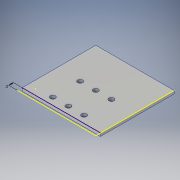
# Autodesk Inventor part: nhk20
Saved by Autodesk Inventor 2019 (Build 230136000, 136)
## iProperties
Created: 2022-02-15
Part Number: nhk20
Material: アルミニウム 6061
Document SubType Name: Sheet Metal
Designer: yuta
Density: 2.7 g/cm^3
Sheet Metal Rule: Default_mm
Appearance: アルミニウム - フラット
Mass: 12.461 g
Surface Area: 51.1627 cm^2
Volume: 4.61518 cm^3
Author: yuta
Autodesk Inventor part; units mm, degrees
ref_plane "YZ Plane" through (0, 0, 0) normal (1, 0, 0) x (0, 1, 0)
ref_plane "XZ Plane" through (0, 0, 0) normal (0, 1, 0) x (-1, 0, 0)
ref_plane "XY Plane" through (0, 0, 0) normal (0, 0, 1) x (1, 0, 0)
sketch "スケッチ1" plane through (0, 0, 0) normal (0, 1, 0) x (-1, 0, 0)
  line L0 (5.0263, 6.4044) -> (-44.9737, 6.4044)
  line L1 (-44.9737, 6.4044) -> (-44.9737, -43.5956)
  line L2 (-44.9737, -43.5956) -> (5.0263, -43.5956)
  line L3 (5.0263, -43.5956) -> (5.0263, 6.4044)
  point P0 (0, 0)
  dimension "d0" = 50
  dimension "d1" = 50
  constraints: 8 end point, 2 parallel, 1 horizontal, 1 perpendicular
  measures "d0" distance of L2.end L1.end
  measures "d1" distance of L1.end L0.end
extrude "押し出し1" add sketch "スケッチ1" along normal blind 2
sketch "スケッチ2" plane through (0, 2, 0) normal (0, 1, 0) x (1, 0, 0)
  circle A0 centre (19.9737, 1.0956) radius 1.5
  line L0 (-5.0263, -6.4044) -> (44.9737, -6.4044) projected
  line L1 (-5.0263, 43.5956) -> (-5.0263, -6.4044) projected
  circle A1 centre (9.9737, 1.0956) radius 1.5
  circle A2 centre (29.9737, 1.0956) radius 1.5
  circle A3 centre (9.9737, 18.5956) radius 1.5
  circle A4 centre (19.9737, 18.5956) radius 1.5
  circle A5 centre (29.9737, 18.5956) radius 1.5
  point P0 (0, 0)
  dimension "d4" = 3
  dimension "d5" = 7.5
  dimension "d6" = 25
  dimension "d7" = 3
  dimension "d8" = 3
  dimension "d9" = 10
  dimension "d10" = 10
  dimension "d11" = 3
  dimension "d12" = 17.5
  dimension "d13" = 3
  dimension "d14" = 3
  dimension "d15" = 10
  dimension "d16" = 10
  dimension "d17" = 17.5
  constraints: 6 centre point
  measures "d4" diameter of A0
  measures "d5" distance from line of A0.centre L0
  measures "d6" distance from line of L1 A0.centre
  measures "d7" diameter of A1
  measures "d8" diameter of A2
  measures "d9" distance of A1.centre A0.centre
  measures "d10" distance of A2.centre A0.centre
  measures "d11" diameter of A3
  measures "d12" distance of A1.centre A3.centre
  measures "d13" diameter of A4
  measures "d14" diameter of A5
  measures "d15" distance of A4.centre A3.centre
  measures "d16" distance of A5.centre A4.centre
  measures "d17" distance of A2.centre A5.centre
hole "穴1" at (9.9737, 2, -1.0956) at (19.9737, 2, -1.0956) at (29.9737, 2, -1.0956) at (9.9737, 2, -18.5956) at (19.9737, 2, -18.5956) at (29.9737, 2, -18.5956) direction (0, -1, 0) diameter 3 depth 2
sketch "スケッチ3" plane through (0, 2, 0) normal (0, 1, 0) x (1, 0, 0)
  line L0 (-4.9253, -3.4044) -> (44.9737, -3.4044)
  line L1 (44.9737, -6.4044) -> (44.9737, 43.5956) projected
  line L2 (-5.0263, -6.4044) -> (44.9737, -6.4044) projected
  point P0 (0, 0)
  dimension "d25" = 3
  constraints: 2 end point, 1 horizontal, 1 point on line
  measures "d25" distance between parallel lines of L2 L0
sketch "スケッチ4" plane through (0, 2, 0) normal (0, 1, 0) x (1, 0, 0)
  line L0 (-5.0263, 43.5956) -> (-5.0263, -6.4044) projected
  line L1 (-5.0263, -6.4044) -> (44.9737, -6.4044) projected
  line L2 (-5.0263, -6.4044) -> (44.9737, -6.4044)
  line L3 (44.9737, -6.4044) -> (44.9737, -3.4044)
  line L4 (44.9737, -6.4044) -> (44.9737, 43.5956) projected
  line L5 (44.9737, -3.4044) -> (-5.0263, -3.4044)
  line L6 (-5.0263, -3.4044) -> (-5.0263, -6.4044)
  point P0 (0, 0)
  dimension "d26" = 3
  constraints: 8 end point, 2 perpendicular, 1 horizontal, 1 point on line
  measures "d26" distance of L1.end L3.end
extrude "押し出し2" cut sketch "スケッチ4" against normal blind 10
sketch "スケッチ5" plane through (0, 2, 0) normal (0, 1, 0) x (1, 0, 0)
  circle A0 centre (9.9737, 1.0956) radius 1.6
  line L0 (-5.0263, -3.4044) -> (44.9737, -3.4044) projected
  circle A1 centre (9.9737, 18.5956) radius 1.5 projected
  circle A2 centre (9.9737, 18.5956) radius 1.6
  circle A3 centre (19.9737, 18.5956) radius 1.6
  circle A4 centre (19.9737, 1.0956) radius 1.6
  circle A5 centre (29.9737, 18.5956) radius 1.6
  circle A6 centre (29.9737, 1.0956) radius 1.6
  line L1 (-5.0263, 43.5956) -> (-5.0263, -3.4044) projected
  point P0 (0, 0)
  dimension "d29" = 3.2
  dimension "d30" = 4.5
  dimension "d32" = 3.2
  dimension "d33" = 3.2
  dimension "d34" = 3.2
  dimension "d35" = 3.2
  dimension "d36" = 3.2
  dimension "d37" = 4.5
  dimension "d38" = 17.5
  dimension "d39" = 17.5
  dimension "d40" = 17.5
  dimension "d41" = 4.5
  dimension "d42" = 10
  dimension "d43" = 10
  dimension "d44" = 10
  dimension "d45" = 15
  dimension "d46" = 15
  dimension "d47" = 10
  constraints: 6 centre point, 1 coincident
  measures "d29" diameter of A0
  measures "d30" distance from line of L0 A0.centre
  measures "d32" diameter of A2
  measures "d33" diameter of A3
  measures "d34" diameter of A4
  measures "d35" diameter of A5
  measures "d36" diameter of A6
  measures "d37" distance from line of L0 A4.centre
  measures "d38" distance of A1.centre A0.centre
  measures "d39" distance of A4.centre A3.centre
  measures "d40" distance of A6.centre A5.centre
  measures "d41" distance from line of L0 A6.centre
  measures "d42" distance of A3.centre A1.centre
  measures "d43" distance of A5.centre A3.centre
  measures "d44" distance of A4.centre A0.centre
  measures "d45" distance from line of L1 A1.centre
  measures "d46" distance from line of L1 A0.centre
  measures "d47" distance of A4.centre A6.centre
hole "穴2" at (9.9737, 2, -1.0956) at (19.9737, 2, -1.0956) at (29.9737, 2, -1.0956) at (29.9737, 2, -18.5956) at (19.9737, 2, -18.5956) at (9.9737, 2, -18.5956) direction (0, -1, 0) diameter 3.2 depth 3
equation "\"BendRadius\" = Thickness"
equation "\"BendReliefWidth\" = Thickness"
equation "\"BendReliefDepth\" = 0.5 * Thickness"
equation "\"CornerReliefSize\" = 4 * Thickness"
equation "\"MinimumRemnant\" = 2 * Thickness"
equation "\"TransitionRadius\" = BendRadius"
equation "\"JacobiRadiusSize\" = BendRadius"
equation "\"GapSize\" = Thickness"
equation "\"Thickness\" = 0.5"
